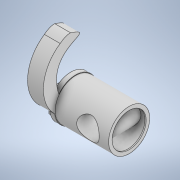
# Autodesk Inventor part: L-turning-knob
Saved by Autodesk Inventor 2020.2 (Build 242310000, 310)
## iProperties
Company: MGDesign (Mammbo Group)
Created: 2020-03-26
Part Number: L-turning-knob
Material: Generic
Document SubType Name: Modeling
Designer: Isaac Ramonet
Density: 1 g/cm^3
Appearance: Default
Author: Isaac Ramonet
Title: R turning knob
Autodesk Inventor part; units mm, degrees
ref_plane "YZ Plane" through (0, 0, 0) normal (1, 0, 0) x (0, 1, 0)
ref_plane "XZ Plane" through (0, 0, 0) normal (0, 1, 0) x (-1, 0, 0)
ref_plane "XY Plane" through (0, 0, 0) normal (0, 0, 1) x (1, 0, 0)
sketch "Sketch1" plane through (0, 0, 0) normal (1, 0, 0) x (0, 1, 0)
  circle A0 centre (0, 0) radius 8.45
  dimension "d0" = 16.9
  constraints: 1 centre point, 1 coincident
  measures "d0" diameter of A0
extrude "Extrusion1" add sketch "Sketch1" along normal blind 13.5 and the other way blind 8.5
sketch "Sketch2" plane through (13.5, 0, 0) normal (1, 0, 0) x (0, 0, -1)
  circle A0 centre (0, 0) radius 7.725
  circle A1 centre (0, 0) radius 9.725
  dimension "d3" = 2
  dimension "d4" = 19.45
  constraints: 2 centre point, 2 coincident
  measures "d3" radial gap between concentric circles of A0 A1
  measures "d4" diameter of A1
extrude "Extrusion2" cut sketch "Sketch2" against normal blind 21.5 contours A0
sketch "Sketch3" plane through (0, 0, 0) normal (0, 0, 1) x (1, 0, 0)
  circle A0 centre (0, 0) radius 5.625
  dimension "d7" = 11.25
  constraints: 1 centre point, 1 coincident
  measures "d7" diameter of A0
extrude "Extrusion3" add sketch "Sketch3" along normal mid plane 18
sketch "Sketch4" plane through (0, 0, 0) normal (0, 0, 1) x (1, 0, 0)
  circle A0 centre (0, 0) radius 4.625
  dimension "d10" = 9.25
  constraints: 1 centre point, 1 coincident
  measures "d10" diameter of A0
extrude "Extrusion5" cut sketch "Sketch4" along normal mid plane 100
sketch "Sketch5" plane through (13.5, 0, 0) normal (1, 0, 0) x (0, 0, -1)
  circle A0 centre (0, 0) radius 8.675
  dimension "d15" = 17.35
  constraints: 1 centre point, 1 coincident
  measures "d15" diameter of A0
extrude "Extrusion6" add sketch "Sketch5" along normal blind 2
sketch "Sketch6" plane through (15.5, 0, 0) normal (1, 0, 0) x (0, 0, -1)
  line L0 (-4.5122, 2.7901) -> (4.4929, 2.7901)
  line L1 (4.5692, -6.1957) -> (-4.5122, -6.1957)
  circle A0 centre (0, 0) radius 8.45 projected
  line L2 (0, 8.45) -> (0, 3.958)
  arc A1 (-6.3756, 23.0304) -> (-4.5122, -3.8079) centre (2.1717, 10.14) ccw
  spline S0 degree 4 poles (-4.5122, 1.1452) (-5.6426, 2.0969) (-5.737, 1.2194) (-16.5677, 25.1311) (9.5845, 20.6894) (-2.1134, 24.7257) knots 0 0 0 0 0 0.341326 1 1 1 1 1
  spline S1 degree 2 poles (-6.3756, 23.0304) (-3.3857, 25.3291) (-1.0628, 24.5204) knots 0 0 0 1 1 1
  line L3 (4.5122, -6.1957) -> (4.5122, 2.7901)
  line L4 (-4.5122, -6.1957) -> (-4.5122, -3.8079)
  line L5 (-4.5122, 1.1452) -> (-4.5122, 2.7901)
  line L6 (-1.0193, -1.7956) -> (-8.0051, 4.086) construction
  arc A2 (-2.1896, -1.5079) -> (-7.5222, 2.9819) centre (-12.0159, -7.7671) ccw construction
  line L7 (4.5122, 2.7901) -> (4.4929, 2.7901)
  point P0 (0.6384, 21.8139)
  point P1 (-3.2364, 24.6304)
  point P2 (-2.1134, 24.7257)
  point P3 (-8.3671, -1.1804)
  point P4 (-6.8647, 4.9273)
  constraints: 16 end point, 4 point on circle, 2 centre point, 2 horizontal, 2 midpoint, 2 symmetric about line, 1 parallel, 1 vertical, 15 other
extrude "Extrusion7" add sketch "Sketch6" along normal blind 4.5 and the other way blind 2 contours L0 L7 L3 L1 L4 A1 A0 S0 L5 | A0 A1 S1 S0 picked at (1.4976, -2.4045)
sketch "Sketch7" plane through (-8.5, 0, 0) normal (-1, 0, 0) x (0, 0, 1)
  circle A0 centre (0, 0) radius 8.45
  circle A1 centre (0, 0) radius 11.1999
  dimension "d23" = 16.9
  constraints: 2 centre point, 2 coincident
  measures "d23" diameter of A0
extrude "Extrusion8" cut sketch "Sketch7" against normal blind 17.75
mirror "Mirror1" about plane through (0, 0, 0) normal (1, 0, 0) remove original yes
sketch "Sketch8" plane through (8.5, 0, 0) normal (1, 0, 0) x (0, 0, -1)
  circle A0 centre (0, 0) radius 7.0092
  constraints: 1 centre point, 1 coincident
extrude "Extrusion9" cut sketch "Sketch8" against normal blind 2
body "Solid1"
